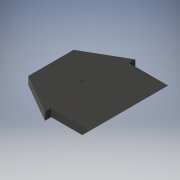
# Autodesk Inventor part: HA02
Saved by Autodesk Inventor 2017 (Build 210142000, 142)
## iProperties
Created: 2018-10-18
Part Number: HA02
Material: ABS Plastic
Document SubType Name: Modeling
Designer: Dell
Density: 1.06 g/cm^3
Appearance: Smooth - Black
Author: Dell
Autodesk Inventor part; units mm, degrees
ref_plane "XZ Plane" through (0, 0, 0) normal (0, 1, 0) x (-1, 0, 0)
ref_plane "XY Plane" through (0, 0, 0) normal (0, 0, 1) x (1, 0, 0)
sketch "Sketch1" plane through (0, 0, 0) normal (0, 0, 1) x (1, 0, 0)
  line L0 (0, 0) -> (100, 0)
  line L1 (100, 0) -> (100, 25)
  line L2 (100, 25) -> (0, 25)
  line L3 (0, 25) -> (0, 0)
  line L4 (0, 25) -> (115.2078, 140.2078)
  line L5 (100, 0) -> (177.7078, 77.7078)
  line L6 (151.2922, 176.2922) -> (200.5844, 163.0844)
  line L7 (200.5844, 163.0844) -> (213.7922, 113.7922)
  line L8 (213.7922, 113.7922) -> (177.7078, 77.7078)
  line L9 (177.7078, 77.7078) -> (128.4156, 90.9156)
  line L10 (128.4156, 90.9156) -> (115.2078, 140.2078)
  line L11 (115.2078, 140.2078) -> (151.2922, 176.2922)
  circle A0 centre (164.5, 127) radius 4
  dimension "d0" = 100
  dimension "d1" = 25
  dimension "d6" = 8
  dimension "d8" = 45
  dimension "d15" = 127
  constraints: 24 end point, 2 collinear, 2 parallel, 1 centre point, 1 coincident, 1 horizontal, 1 perpendicular, 13 other
  measures "d0" distance of L2.end L1.end
  measures "d1" distance of L1.end L0.end
  measures "d6" diameter of A0
  measures "d8" angle of L2 L4
  measures "d15" distance from line of L0 point (164.5, 127)
extrude "Extrusion1" add sketch "Sketch1" along normal blind 20
sketch "Sketch2" plane through (0, 0, 20) normal (0, 0, 1) x (1, 0, 0)
  line L0 (0, 25) -> (0, 0) projected
  line L1 (0, 0) -> (100, 0) projected
  line L2 (0, 25) -> (100, 25)
  line L3 (100, 25) -> (100, 0)
  line L4 (100, 0) -> (0, 0)
  line L5 (0, 0) -> (0, 25)
  line L6 (100, 25) -> (125, 25)
  line L7 (100, 0) -> (213.7922, 113.7922) projected
  line L8 (100, 0) -> (125, 25)
  constraints: 12 end point, 2 horizontal, 2 parallel, 1 perpendicular, 1 point on line
extrude "Extrusion2" add sketch "Sketch2" along normal blind 250
sketch "Sketch4" plane through (0, 0, 270) normal (0, 0, 1) x (1, 0, 0)
  line L0 (0, 25) -> (125, 25) projected
  line L1 (125, 25) -> (213.7922, 113.7922) projected
  line L2 (213.7922, 113.7922) -> (200.5844, 163.0844) projected
  line L3 (200.5844, 163.0844) -> (151.2922, 176.2922) projected
  line L4 (151.2922, 176.2922) -> (0, 25) projected
  circle A0 centre (164.5, 127) radius 4 projected
  line L5 (100, 0) -> (125, 25) projected
  line L6 (125, 25) -> (0, 25) projected
  line L7 (0, 25) -> (0, 0) projected
  line L8 (0, 0) -> (100, 0) projected
extrude "Extrusion3" add sketch "Sketch4" along normal blind 20
sketch "Sketch5" plane through (0, 0, 0) normal (0, -1, 0) x (1, 0, 0)
  line L0 (0, 0) -> (100, 0) projected
  line L1 (100, 0) -> (100, 290) projected
  line L2 (0, 290) -> (100, 290) projected
  line L3 (0, 0) -> (0, 290) projected
  line L4 (0, 0) -> (-125.5737, 72.5)
  line L5 (-125.5737, 72.5) -> (-125.5737, 217.5)
  line L6 (-125.5737, 217.5) -> (0, 290)
  line L7 (0, 290) -> (125.5737, 217.5)
  line L8 (125.5737, 217.5) -> (125.5737, 72.5)
  line L9 (125.5737, 72.5) -> (0, 0)
  point P0 (0, 145)
  constraints: 12 end point, 13 other
extrude "Extrusion4" add sketch "Sketch5" against normal blind 25 contours L4 L5 L6 L3
sketch "Sketch6" plane through (0, 25, 20) normal (0, 1, 0) x (1, 0, 0)
  line L0 (100, 20) -> (100, -270) projected
  circle A0 centre (-24.528, -125) radius 3
  circle A1 centre (-31.528, -125) radius 1.5
  circle A2 centre (-21.028, -131.0622) radius 1.5
  circle A3 centre (-21.028, -118.9378) radius 1.5
  point P0 (0, 20)
  point P1 (100, -125)
  dimension "d18" = 6
  dimension "d19" = 124.528
  dimension "d20" = 3
  dimension "d21" = 7
  dimension "d24" = 360
  constraints: 4 centre point, 2 horizontal alignment, 1 midpoint, 7 other
  measures "d18" diameter of A0
  measures "d19" distance from line of L0 A0.centre
  measures "d20" diameter of A1
  measures "d21" distance of A1.centre A0.centre
extrude "Extrusion5" cut sketch "Sketch6" against normal through all
sketch "Sketch7" plane through (100, 0, 0) normal (0, -1, 0) x (1, 0, 0)
  circle A0 centre (-124.528, 145) radius 3 projected
  circle A1 centre (-124.528, 145) radius 12
  point P0 (-100, 0)
  dimension "d28" = 24
  constraints: 1 centre point, 1 coincident
  measures "d28" diameter of A1
extrude "Extrusion6" cut sketch "Sketch7" against normal blind 5
sketch "Sketch8" plane through (0, 0, 270) normal (0, 0, -1) x (-1, 0, 0)
  circle A0 centre (-164.5, 127) radius 4 projected
  circle A1 centre (-164.5, 127) radius 12.5
  point P0 (0, 0)
  dimension "d31" = 25
  constraints: 1 centre point, 1 coincident
  measures "d31" diameter of A1
extrude "Extrusion7" cut sketch "Sketch8" against normal blind 7
sketch "Sketch10" plane through (164.5, 127, 277) normal (0, 0, -1) x (-1, 0, 0)
  circle A0 centre (7, 0) radius 2
  circle A1 centre (0, 0) radius 4 projected
  circle A2 centre (-3.5, 6.0622) radius 2
  circle A3 centre (-3.5, -6.0622) radius 2
  point P0 (164.5, -127)
  dimension "d34" = 4
  dimension "d37" = 360
  dimension "d39" = 7
  constraints: 3 centre point, 1 horizontal alignment, 7 other
  measures "d34" diameter of A0
  measures "d39" distance of A0.centre A1.centre
extrude "Extrusion8" cut sketch "Sketch10" against normal through all
sketch "Sketch11" plane through (0, 0, 290) normal (0, 0, 1) x (1, 0, 0)
  circle A0 centre (168, 133.0622) radius 2 projected
  circle A1 centre (164.5, 127) radius 4 projected
  circle A2 centre (168, 133.0622) radius 4
  circle A3 centre (157.5, 127) radius 4
  circle A4 centre (168, 120.9378) radius 4
  point P0 (0, 0)
  dimension "d42" = 8
  dimension "d45" = 360
  constraints: 3 centre point, 1 coincident, 7 other
  measures "d42" diameter of A2
extrude "Extrusion9" cut sketch "Sketch11" against normal blind 3 contours A0 | A1 A4 A3 A2 | A2 A1 | A1 A2 | A4 A1 | A1 A4 | A3 A1 | A1 A3
ref_plane "Work Plane1" through (164.5, 127, 270) normal (1, 0, 0) x (0, 0, 1)
sketch "Sketch12" plane through (164.5, 127, 270) normal (1, 0, 0) x (0, 0, 1)
  line L0 (17, -1.9365) -> (17, 1.9365) projected
  line L1 (17, 1.9365) -> (20, 1.9365) projected
  line L2 (20, 3.9993) -> (20, 1.9365) projected
  line L3 (20, 3.9993) -> (17, 3.9993) projected
  line L4 (17, 3.9993) -> (17, 2.0628) projected
  line L5 (17, 2.0628) -> (20, 2.0628) projected
  line L6 (20, -2.0628) -> (20, 2.0628) projected
  line L7 (20, -2.0628) -> (17, -2.0628) projected
  line L8 (17, -2.0628) -> (17, -3.9993) projected
  line L9 (17, -3.9993) -> (20, -3.9993) projected
  line L10 (20, -1.9365) -> (20, -3.9993) projected
  line L11 (20, -1.9365) -> (17, -1.9365) projected
  line L12 (7, 4) -> (7, -4) projected
  line L13 (7, -12.5) -> (7, 12.5) projected
  line L14 (0, -12.5) -> (0, 12.5) projected
  circle A0 centre (3.5, 0) radius 2
  line L15 (0, -12.5) -> (7, -12.5) projected
  point P0 (-270, 127)
  point P1 (7, 0)
  point P2 (3.5, -12.5)
  dimension "d50" = 4
  constraints: 2 midpoint, 1 centre point, 1 horizontal alignment, 1 vertical alignment
  measures "d50" diameter of A0
extrude "Extrusion10" cut sketch "Sketch12" along normal through all contours A0
sketch "Sketch13" plane through (0, 0, 290) normal (0, 0, 1) x (1, 0, 0)
  line L0 (100, 0) -> (213.7922, 113.7922) projected
  line L1 (213.7922, 113.7922) -> (200.5844, 163.0844) projected
  line L2 (200.5844, 163.0844) -> (151.2922, 176.2922) projected
  line L3 (151.2922, 176.2922) -> (0, 25) projected
  line L4 (0, 25) -> (0, 0) projected
  line L5 (0, 0) -> (100, 0) projected
  arc A0 (161, 128.9365) -> (161, 125.0635) centre (157.5, 127) ccw projected
  arc A1 (164.5729, 130.9993) -> (161, 128.9365) centre (164.5, 127) ccw projected
  arc A2 (167.9271, 129.0628) -> (164.5729, 130.9993) centre (168, 133.0622) ccw projected
  arc A3 (167.9271, 124.9372) -> (167.9271, 129.0628) centre (164.5, 127) ccw projected
  arc A4 (164.5729, 123.0007) -> (167.9271, 124.9372) centre (168, 120.9378) ccw projected
  arc A5 (161, 125.0635) -> (164.5729, 123.0007) centre (164.5, 127) ccw projected
extrude "Extrusion11" cut sketch "Sketch13" against normal blind 20 contours L5 L4 L3 L2 L1 L0 | A1 A2 A3 A4 A5 A0
sketch "Sketch14" plane through (0, 0, 0) normal (0, 0, -1) x (-1, 0, 0)
  circle A0 centre (-164.5, 127) radius 4 projected
  line L0 (0, 0) -> (-100, 0) projected
  line L1 (0, 25) -> (0, 0) projected
  line L2 (-151.2922, 176.2922) -> (0, 25) projected
  line L3 (-200.5844, 163.0844) -> (-151.2922, 176.2922) projected
  line L4 (-213.7922, 113.7922) -> (-200.5844, 163.0844) projected
  line L5 (-100, 0) -> (-213.7922, 113.7922) projected
extrude "Extrusion12" cut sketch "Sketch14" against normal blind 20
sketch "Sketch15" plane through (0, 0, 20) normal (0, 0, -1) x (-1, 0, 0)
  circle A0 centre (-90, 12.5) radius 2.5
  circle A1 centre (-15, 12.5) radius 2.5
  line L0 (-90, 12.5) -> (-15, 12.5) construction
  line L1 (0, 0) -> (-100, 0) projected
  dimension "d57" = 5
  dimension "d58" = 5
  dimension "d59" = 75
  dimension "d60" = 12.5
  dimension "d61" = 10
  constraints: 2 centre point, 2 end point, 1 horizontal
  measures "d57" diameter of A0
  measures "d58" diameter of A1
  measures "d59" distance of L0.start L0.end
  measures "d60" distance between parallel lines of L1 L0
  measures "d61" horizontal distance of L1.end L0.start
extrude "Extrusion13" cut sketch "Sketch15" against normal through all
body "Solid1"
